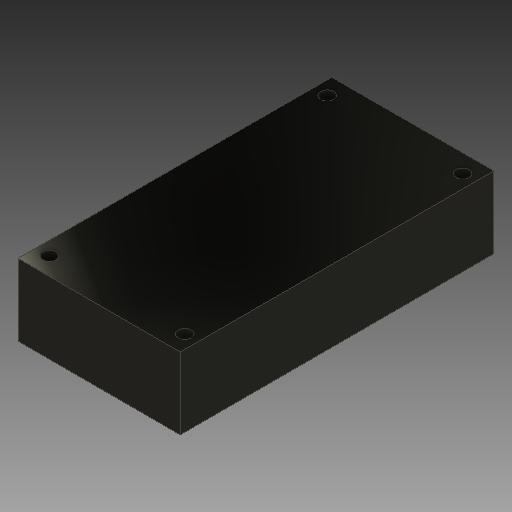
# Autodesk Inventor part: boost
Saved by Autodesk Inventor 2020 (Build 240168000, 168)
## iProperties
Created: 2024-09-30
Part Number: boost
Material: Типовые
Document SubType Name: Modeling
Designer: Ivan
Density: 1 g/cm^3
Appearance: Оружейный металл
Mass: 40.0916 g
Surface Area: 90.1304 cm^2
Volume: 40.0916 cm^3
Author: Ivan
Autodesk Inventor part; units mm, degrees
ref_plane "YZ Plane" through (0, 0, 0) normal (1, 0, 0) x (0, 1, 0)
ref_plane "XZ Plane" through (0, 0, 0) normal (0, 1, 0) x (-1, 0, 0)
ref_plane "XY Plane" through (0, 0, 0) normal (0, 0, 1) x (1, 0, 0)
sketch "Эскиз1" plane through (0, 0, 0) normal (0, 1, 0) x (-1, 0, 0)
  line L0 (18.1, 35) -> (-18.1, 35)
  line L1 (-18.1, 35) -> (-18.1, -35)
  line L2 (-18.1, -35) -> (18.1, -35)
  line L3 (18.1, -35) -> (18.1, 35)
  line L4 (18.1, 35) -> (-18.1, -35) construction
  line L5 (15.1, 31) -> (15.1, -31)
  line L6 (0, 0) -> (5, 0) construction
  circle A0 centre (15.1, 31) radius 1.5
  line L7 (0, 0) -> (0, 5) construction
  line L8 (0, 0) -> (3, -3) construction
  circle A1 centre (-15.1, 31) radius 1.5
  circle A2 centre (15.1, -31) radius 1.5
  circle A3 centre (-15.1, -31) radius 1.5
  point P0 (15.1, 0)
  point P1 (-15.5, 0)
  dimension "d0" = 36.2
  dimension "d1" = 70
  dimension "d2" = 4
  dimension "d3" = 3
  dimension "d4" = 3
  constraints: 18 end point, 4 centre point, 3 parallel, 3 symmetric about line, 2 coincident, 2 horizontal, 2 midpoint, 2 perpendicular, 2 point on line, 1 vertical, 3 other
  measures "d0" distance of L2.end L1.end
  measures "d1" distance of L1.end L0.end
  measures "d2" distance from line of L0 L5.start
  measures "d3" distance from line of L3 point (15.1, 0)
  measures "d4" diameter of A0
extrude "Выдавливание1" add sketch "Эскиз1" along normal blind 16
